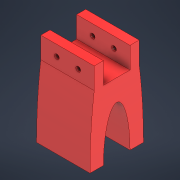
# Autodesk Inventor part: Arch
Saved by Autodesk Inventor 2022 (Build 260153000, 153)
## iProperties
Created: 2022-04-07
Part Number: Arch
Material: ABS Plastic
Document SubType Name: Modeling
Designer: Sergei
Density: 1.06 g/cm^3
Appearance: Light Red
Author: Sergei
Autodesk Inventor part; units mm, degrees
ref_plane "YZ Plane" through (0, 0, 0) normal (1, 0, 0) x (0, 1, 0)
ref_plane "XZ Plane" through (0, 0, 0) normal (0, 1, 0) x (-1, 0, 0)
ref_plane "XY Plane" through (0, 0, 0) normal (0, 0, 1) x (1, 0, 0)
sketch "Sketch1" plane through (0, 0, 0) normal (1, 0, 0) x (0, 1, 0)
  ellipse E0 centre (0, -25) end of major axis (45, -25) minor radius 12.5 (0, -37.5) -> (0, -12.5) ccw
  ellipse E1 centre (0, -25) end of major axis (120, -25) minor radius 25 (0, -50) -> (0, 0) ccw
  line L0 (65, -3.9852) -> (65, -46.0148)
  line L1 (0, -37.5) -> (0, -50)
  line L2 (0, -12.5) -> (0, 0)
  point P0 (0, -43.75)
  point P1 (0, -6.25)
  dimension "d23" = 45
  dimension "d25" = 120
  dimension "d18" = 50
  dimension "d22" = 25
  dimension "d24" = 65
  constraints: 6 end point, 3 vertical, 2 midpoint, 2 vertical alignment, 1 coincident, 10 other
  measures "d18" distance of L2.end L1.end
  measures "d22" distance of L2.start L1.start
  measures "d24" distance between parallel lines of L1 L0
extrude "Extrusion1" add sketch "Sketch1" along normal blind 50 contours E0 L2 E1 L0 L1
sketch "Sketch3" plane through (0, 65, -3.9852) normal (0, 1, 0) x (1, 0, 0)
  line L0 (0, 42.0297) -> (0, 0) projected
  line L1 (0, 0) -> (50, 0) projected
  line L2 (50, 42.0297) -> (50, 0) projected
  line L3 (0, 42.0297) -> (50, 42.0297) projected
  line L4 (0, 33.5148) -> (0, 8.5148) projected
  line L5 (50, 0) -> (0, 0)
  line L6 (0, 0) -> (0, 8.5148)
  line L7 (0, 8.5148) -> (50, 8.5148)
  line L8 (50, 8.5148) -> (50, 0)
  line L9 (0, 42.0297) -> (50, 42.0297)
  line L10 (50, 42.0297) -> (50, 33.5148)
  line L11 (50, 33.5148) -> (0, 33.5148)
  line L12 (0, 33.5148) -> (0, 42.0297)
  point P0 (0, -3.9852)
  point P1 (0, 33.5148)
  dimension "d26" = 25
  dimension "d27" = 8.5148
  dimension "d28" = 8.5148
  constraints: 16 end point, 4 parallel, 2 horizontal, 2 perpendicular, 2 point on line
  measures "d26" distance between parallel lines of L11 L7
  measures "d27" distance between parallel lines of L7 L1
  measures "d28" distance between parallel lines of L3 L11
extrude "Extrusion3" add sketch "Sketch3" along normal blind 20 contours L3 L2 L11 L0 | L7 L2 L1 L0
sketch "Sketch4" plane through (50, 65, -46.0148) normal (0, 0, -1) x (-1, 0, 0)
  line L0 (50, 0) -> (0, 0) projected
  line L1 (50, 0) -> (50, 20) projected
  line L2 (0, 20) -> (50, 20) projected
  line L3 (0, 0) -> (0, 20) projected
  line L4 (0, 0) -> (0, 20) projected
  line L5 (0, 10) -> (50, 10)
  circle A0 centre (15, 10) radius 2.25
  circle A1 centre (35, 10) radius 2.25
  point P0 (50, -65)
  dimension "d31" = 4.5
  dimension "d32" = 4.5
  dimension "d33" = 20
  dimension "d34" = 15
  dimension "d35" = 15
  constraints: 2 centre point, 2 end point, 2 midpoint, 2 point on line
  measures "d31" diameter of A0
  measures "d32" diameter of A1
  measures "d33" distance of A1.centre A0.centre
  measures "d34" distance of L5.start A0.centre
  measures "d35" distance of L5.end A1.centre
extrude "Extrusion4" cut sketch "Sketch4" against normal through all contours A1 L5 | L5 A1 | A0 L5 | L5 A0
sketch "Sketch5" plane through (0, 0, -12.5) normal (0, -1, 0) x (1, 0, 0)
  line L0 (0, 12.5) -> (0, 0) projected
  line L1 (0, 0) -> (50, 0) projected
  line L2 (50, 12.5) -> (50, 0) projected
  line L3 (0, 12.5) -> (50, 12.5) projected
  line L4 (0, -25) -> (0, -37.5) projected
  line L5 (0, -37.5) -> (50, -37.5) projected
  line L6 (50, -25) -> (50, -37.5) projected
  line L7 (0, -25) -> (50, -25) projected
  line L8 (50, 8.5148) -> (50, 12.5) projected
  line L9 (0, -25) -> (0, -37.5) projected
  line L10 (50, 12.5) -> (0, -37.5)
  line L11 (5.7, 6.8) -> (44.3, 6.8)
  line L12 (44.3, 6.8) -> (44.3, -31.8)
  line L13 (44.3, -31.8) -> (5.7, -31.8)
  line L14 (5.7, -31.8) -> (5.7, 6.8)
  line L15 (5.7, 6.8) -> (44.3, -31.8) construction
  line L16 (44.3, 6.8) -> (5.7, -31.8) construction
  line L17 (44.3, 3.3) -> (41.2689, 5.05)
  line L18 (41.2689, 5.05) -> (41.2689, 8.55)
  line L19 (41.2689, 8.55) -> (44.3, 10.3)
  line L20 (44.3, 10.3) -> (47.3311, 8.55)
  line L21 (47.3311, 8.55) -> (47.3311, 5.05)
  line L22 (47.3311, 5.05) -> (44.3, 3.3)
  line L23 (41.2689, -33.55) -> (41.2689, -30.05)
  line L24 (41.2689, -30.05) -> (44.3, -28.3)
  line L25 (44.3, -28.3) -> (47.3311, -30.05)
  line L26 (47.3311, -30.05) -> (47.3311, -33.55)
  line L27 (47.3311, -33.55) -> (44.3, -35.3)
  line L28 (44.3, -35.3) -> (41.2689, -33.55)
  line L29 (8.7311, -30.05) -> (8.7311, -33.55)
  line L30 (8.7311, -33.55) -> (5.7, -35.3)
  line L31 (5.7, -35.3) -> (2.6689, -33.55)
  line L32 (2.6689, -33.55) -> (2.6689, -30.05)
  line L33 (2.6689, -30.05) -> (5.7, -28.3)
  line L34 (5.7, -28.3) -> (8.7311, -30.05)
  line L35 (8.7311, 8.55) -> (8.7311, 5.05)
  line L36 (8.7311, 5.05) -> (5.7, 3.3)
  line L37 (5.7, 3.3) -> (2.6689, 5.05)
  line L38 (2.6689, 5.05) -> (2.6689, 8.55)
  line L39 (2.6689, 8.55) -> (5.7, 10.3)
  line L40 (5.7, 10.3) -> (8.7311, 8.55)
  point P0 (25, -12.5)
  dimension "d38" = 38.6
  dimension "d39" = 38.6
  dimension "d40" = 7
  dimension "d41" = 7
  dimension "d42" = 7
  dimension "d43" = 7
  constraints: 62 end point, 4 coincident, 3 midpoint, 3 vertical alignment, 2 parallel, 1 horizontal, 1 perpendicular, 1 vertical, 52 other
  measures "d38" distance of L12.end L13.end
  measures "d39" distance of L11.end L12.end
  measures "d40" distance of L17.start L19.end
  measures "d41" distance of L27.end L24.end
  measures "d42" distance of L30.end L33.end
  measures "d43" distance of L36.end L39.end
extrude "Extrusion5" cut sketch "Sketch5" against normal blind 10 contours L20 L21 L22 L12 L10 | L10 L11 L18 L19 L20 | L37 L38 L39 L40 L35 L11 L14 | L14 L11 L35 L36 | L12 L17 L10 | L10 L17 L18 L11 | L34 L10 L14 | L14 L10 L31 L32 L33 | L34 L29 L13 L10 | L13 L29 L30 L31 L10 | L25 L26 L27 L28 L23 L13 L12 | L12 L13 L23 L24
equation "\"d27\" = d28"
body "Solid1"
